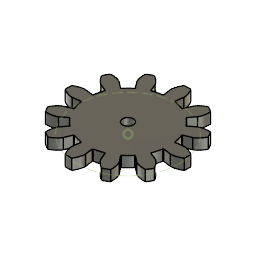
klenn final 1 (Autodesk Fusion 360 archive; units mm, degrees)
design "klenn part_Spur Gear 12 teeth"
description: Spur Gear; Module: 4.0; Num Teeth: 12; Pressure Angle: 14.500000000000002; Backlash: 0.00 mm
part number: 2026-03-30-23-41-15-883
Autodesk Fusion 360 part; units mm, degrees
sketch "Base Circle" plane through (0, 0, 0) normal (0, 0, 1) x (1, 0, 0)
  circle A0 centre (0, 0) radius 19.372
  circle A1 centre (0, 0) radius 2.5
extrude "Extrude1" add sketch "Base Circle" along normal blind 5
sketch "Gear Tooth" plane through (0, 0, 0) normal (0, 0, 1) x (1, 0, 0)
  spline S0 degree 5 poles (23.0196, -3.1605) (23.0336, -3.1625) (23.0617, -3.1659) (23.1038, -3.1698) (23.1603, -3.1727) (23.231, -3.173) (23.302, -3.171) (23.373, -3.1677) (23.4442, -3.1635) (23.5153, -3.1589) (23.5865, -3.1536) (23.6578, -3.1477) (23.7291, -3.1407) (23.8004, -3.1326) (23.8718, -3.1234) (23.9433, -3.1131) (24.0147, -3.102) (24.0862, -3.0901) (24.1576, -3.0775) (24.2291, -3.0643) (24.3005, -3.0505) (24.372, -3.036) (24.4435, -3.0208) (24.5149, -3.0049) (24.5863, -2.9883) (24.6577, -2.9711) (24.7291, -2.9531) (24.8005, -2.9346) (24.8719, -2.9155) (24.9432, -2.8958) (25.0145, -2.8755) (25.0858, -2.8547) (25.157, -2.8332) (25.2282, -2.8112) (25.2993, -2.7887) (25.3705, -2.7656) (25.4415, -2.7419) (25.5126, -2.7177) (25.5835, -2.6929) (25.6545, -2.6677) (25.7254, -2.6419) (25.7962, -2.6156) (25.867, -2.5888) (25.9377, -2.5615) (26.0083, -2.5337) (26.0789, -2.5054) (26.1495, -2.4766) (26.2199, -2.4473) (26.2903, -2.4175) (26.3607, -2.3873) (26.4309, -2.3566) (26.5011, -2.3254) (26.5713, -2.2937) (26.6413, -2.2616) (26.7113, -2.229) (26.7812, -2.196) (26.851, -2.1625) (26.9207, -2.1285) (26.9904, -2.0942) (27.06, -2.0593) (27.1295, -2.024) (27.1989, -1.9883) (27.2682, -1.9522) (27.3374, -1.9156) (27.4065, -1.8786) (27.4756, -1.8411) (27.5445, -1.8033) (27.6134, -1.765) (27.6821, -1.7263) (27.7508, -1.6872) (27.8193, -1.6476) (27.8741, -1.6156) (27.9151, -1.5915) (27.9424, -1.5753) (27.9561, -1.5672) knots 0 0 0 0 0 0 0.01428571 0.02857143 0.04285714 0.05714286 0.07142857 0.08571429 0.1 0.11428571 0.12857143 0.14285714 0.15714286 0.17142857 0.18571429 0.2 0.21428571 0.22857143 0.24285714 0.25714286 0.27142857 0.28571429 0.3 0.31428571 0.32857143 0.34285714 0.35714286 0.37142857 0.38571429 0.4 0.41428571 0.42857143 0.44285714 0.45714286 0.47142857 0.48571429 0.5 0.51428571 0.52857143 0.54285714 0.55714286 0.57142857 0.58571429 0.6 0.61428571 0.62857143 0.64285714 0.65714286 0.67142857 0.68571429 0.7 0.71428571 0.72857143 0.74285714 0.75714286 0.77142857 0.78571429 0.8 0.81428571 0.82857143 0.84285714 0.85714286 0.87142857 0.88571429 0.9 0.91428571 0.92857143 0.94285714 0.95714286 0.97142857 0.98571429 1 1 1 1 1 1
  spline S1 degree 5 poles (23.0196, 3.1605) (23.0336, 3.1625) (23.0617, 3.1659) (23.1038, 3.1698) (23.1603, 3.1727) (23.231, 3.173) (23.302, 3.171) (23.373, 3.1677) (23.4442, 3.1635) (23.5153, 3.1589) (23.5865, 3.1536) (23.6578, 3.1477) (23.7291, 3.1407) (23.8004, 3.1326) (23.8718, 3.1234) (23.9433, 3.1131) (24.0147, 3.102) (24.0862, 3.0901) (24.1576, 3.0775) (24.2291, 3.0643) (24.3005, 3.0505) (24.372, 3.036) (24.4435, 3.0208) (24.5149, 3.0049) (24.5863, 2.9883) (24.6577, 2.9711) (24.7291, 2.9531) (24.8005, 2.9346) (24.8719, 2.9155) (24.9432, 2.8958) (25.0145, 2.8755) (25.0858, 2.8547) (25.157, 2.8332) (25.2282, 2.8112) (25.2993, 2.7887) (25.3705, 2.7656) (25.4415, 2.7419) (25.5126, 2.7177) (25.5835, 2.6929) (25.6545, 2.6677) (25.7254, 2.6419) (25.7962, 2.6156) (25.867, 2.5888) (25.9377, 2.5615) (26.0083, 2.5337) (26.0789, 2.5054) (26.1495, 2.4766) (26.2199, 2.4473) (26.2903, 2.4175) (26.3607, 2.3873) (26.4309, 2.3566) (26.5011, 2.3254) (26.5713, 2.2937) (26.6413, 2.2616) (26.7113, 2.229) (26.7812, 2.196) (26.851, 2.1625) (26.9207, 2.1285) (26.9904, 2.0942) (27.06, 2.0593) (27.1295, 2.024) (27.1989, 1.9883) (27.2682, 1.9522) (27.3374, 1.9156) (27.4065, 1.8786) (27.4756, 1.8411) (27.5445, 1.8033) (27.6134, 1.765) (27.6821, 1.7263) (27.7508, 1.6872) (27.8193, 1.6476) (27.8741, 1.6156) (27.9151, 1.5915) (27.9424, 1.5753) (27.9561, 1.5672) knots 0 0 0 0 0 0 0.01428571 0.02857143 0.04285714 0.05714286 0.07142857 0.08571429 0.1 0.11428571 0.12857143 0.14285714 0.15714286 0.17142857 0.18571429 0.2 0.21428571 0.22857143 0.24285714 0.25714286 0.27142857 0.28571429 0.3 0.31428571 0.32857143 0.34285714 0.35714286 0.37142857 0.38571429 0.4 0.41428571 0.42857143 0.44285714 0.45714286 0.47142857 0.48571429 0.5 0.51428571 0.52857143 0.54285714 0.55714286 0.57142857 0.58571429 0.6 0.61428571 0.62857143 0.64285714 0.65714286 0.67142857 0.68571429 0.7 0.71428571 0.72857143 0.74285714 0.75714286 0.77142857 0.78571429 0.8 0.81428571 0.82857143 0.84285714 0.85714286 0.87142857 0.88571429 0.9 0.91428571 0.92857143 0.94285714 0.95714286 0.97142857 0.98571429 1 1 1 1 1 1
  arc A0 (27.9561, -1.5672) -> (27.9561, 1.5672) centre (0, 0) ccw
  line L0 (19.182, -2.6336) -> (23.0196, -3.1605)
  line L1 (19.182, 2.6336) -> (23.0196, 3.1605)
  line L2 (19.182, -2.6336) -> (19.182, 2.6336)
  point P0 (23.362, -3.168)
  point P1 (23.7088, -3.1425)
  point P2 (24.0583, -3.0946)
  point P3 (24.4097, -3.0279)
  point P4 (24.7627, -2.9443)
  point P5 (25.1168, -2.8453)
  point P6 (25.4717, -2.7315)
  point P7 (25.8272, -2.6038)
  point P8 (26.1829, -2.4626)
  point P9 (26.5385, -2.3084)
  point P10 (26.8939, -2.1415)
  point P11 (27.2488, -1.9622)
  point P12 (27.6029, -1.7707)
  point P13 (23.362, 3.168)
  point P14 (23.7088, 3.1425)
  point P15 (24.0583, 3.0946)
  point P16 (24.4097, 3.0279)
  point P17 (24.7627, 2.9443)
  point P18 (25.1168, 2.8453)
  point P19 (25.4717, 2.7315)
  point P20 (25.8272, 2.6038)
  point P21 (26.1829, 2.4626)
  point P22 (26.5385, 2.3084)
  point P23 (26.8939, 2.1415)
  point P24 (27.2488, 1.9622)
  point P25 (27.6029, 1.7707)
extrude "Extrude2" add sketch "Gear Tooth" along normal blind 5
fillet "Fillet1" radius 0.2 2 edges at (19.192, -2.635, 2.5) (19.192, 2.635, 2.5)
pattern_circular "C-Pattern1" count 12 over 360 about axis through (0, 0, 0) along (0, 0, 1) of "Extrude2", "Fillet1"
sketch "Diametrial Pitch Circle" plane through (0, 0, 0) normal (0, 0, 1) x (1, 0, 0)
  circle A0 centre (0, 0) radius 24 construction

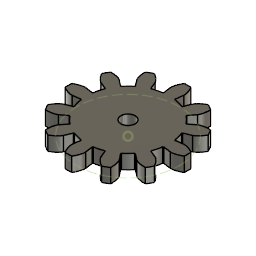
design "klenn part_Spur Gear 12 teeth (1)"
description: Spur Gear; Module: 3.0; Num Teeth: 12; Pressure Angle: 14.500000000000002; Backlash: 0.00 mm
part number: 2026-03-30-23-48-04-964
Autodesk Fusion 360 part; units mm, degrees
sketch "Base Circle" plane through (0, 0, 0) normal (0, 0, 1) x (1, 0, 0)
  circle A0 centre (0, 0) radius 14.529
  circle A1 centre (0, 0) radius 2.5
extrude "Extrude1" add sketch "Base Circle" along normal blind 5
sketch "Gear Tooth" plane through (0, 0, 0) normal (0, 0, 1) x (1, 0, 0)
  spline S0 degree 5 poles (17.2647, -2.3704) (17.2752, -2.3718) (17.2962, -2.3744) (17.3277, -2.3773) (17.3699, -2.3795) (17.4228, -2.3798) (17.4758, -2.3783) (17.529, -2.3758) (17.5822, -2.3727) (17.6355, -2.3692) (17.6887, -2.3653) (17.7421, -2.3609) (17.7954, -2.3557) (17.8488, -2.3497) (17.9023, -2.3428) (17.9557, -2.3351) (18.0092, -2.3268) (18.0627, -2.3179) (18.1162, -2.3085) (18.1697, -2.2986) (18.2232, -2.2883) (18.2768, -2.2775) (18.3303, -2.2661) (18.3838, -2.2542) (18.4373, -2.2418) (18.4908, -2.2289) (18.5443, -2.2155) (18.5978, -2.2016) (18.6513, -2.1873) (18.7048, -2.1726) (18.7582, -2.1574) (18.8116, -2.1418) (18.865, -2.1258) (18.9184, -2.1093) (18.9718, -2.0924) (19.0251, -2.0751) (19.0784, -2.0573) (19.1317, -2.0392) (19.1849, -2.0207) (19.2381, -2.0017) (19.2913, -1.9824) (19.3445, -1.9627) (19.3976, -1.9426) (19.4506, -1.9222) (19.5037, -1.9013) (19.5566, -1.8801) (19.6096, -1.8585) (19.6625, -1.8365) (19.7153, -1.8142) (19.7681, -1.7915) (19.8209, -1.7684) (19.8736, -1.745) (19.9263, -1.7213) (19.9789, -1.6972) (20.0314, -1.6727) (20.084, -1.6479) (20.1364, -1.6228) (20.1888, -1.5973) (20.2411, -1.5714) (20.2934, -1.5453) (20.3456, -1.5188) (20.3978, -1.492) (20.4499, -1.4648) (20.5019, -1.4373) (20.5539, -1.4095) (20.6058, -1.3814) (20.6576, -1.3529) (20.7093, -1.3241) (20.761, -1.295) (20.8127, -1.2656) (20.8642, -1.2359) (20.9054, -1.2118) (20.9362, -1.1937) (20.9568, -1.1815) (20.9671, -1.1754) knots 0 0 0 0 0 0 0.01428571 0.02857143 0.04285714 0.05714286 0.07142857 0.08571429 0.1 0.11428571 0.12857143 0.14285714 0.15714286 0.17142857 0.18571429 0.2 0.21428571 0.22857143 0.24285714 0.25714286 0.27142857 0.28571429 0.3 0.31428571 0.32857143 0.34285714 0.35714286 0.37142857 0.38571429 0.4 0.41428571 0.42857143 0.44285714 0.45714286 0.47142857 0.48571429 0.5 0.51428571 0.52857143 0.54285714 0.55714286 0.57142857 0.58571429 0.6 0.61428571 0.62857143 0.64285714 0.65714286 0.67142857 0.68571429 0.7 0.71428571 0.72857143 0.74285714 0.75714286 0.77142857 0.78571429 0.8 0.81428571 0.82857143 0.84285714 0.85714286 0.87142857 0.88571429 0.9 0.91428571 0.92857143 0.94285714 0.95714286 0.97142857 0.98571429 1 1 1 1 1 1
  spline S1 degree 5 poles (17.2647, 2.3704) (17.2752, 2.3718) (17.2962, 2.3744) (17.3277, 2.3773) (17.3699, 2.3795) (17.4228, 2.3798) (17.4758, 2.3783) (17.529, 2.3758) (17.5822, 2.3727) (17.6355, 2.3692) (17.6887, 2.3653) (17.7421, 2.3609) (17.7954, 2.3557) (17.8488, 2.3497) (17.9023, 2.3428) (17.9557, 2.3351) (18.0092, 2.3268) (18.0627, 2.3179) (18.1162, 2.3085) (18.1697, 2.2986) (18.2232, 2.2883) (18.2768, 2.2775) (18.3303, 2.2661) (18.3838, 2.2542) (18.4373, 2.2418) (18.4908, 2.2289) (18.5443, 2.2155) (18.5978, 2.2016) (18.6513, 2.1873) (18.7048, 2.1726) (18.7582, 2.1574) (18.8116, 2.1418) (18.865, 2.1258) (18.9184, 2.1093) (18.9718, 2.0924) (19.0251, 2.0751) (19.0784, 2.0573) (19.1317, 2.0392) (19.1849, 2.0207) (19.2381, 2.0017) (19.2913, 1.9824) (19.3445, 1.9627) (19.3976, 1.9426) (19.4506, 1.9222) (19.5037, 1.9013) (19.5566, 1.8801) (19.6096, 1.8585) (19.6625, 1.8365) (19.7153, 1.8142) (19.7681, 1.7915) (19.8209, 1.7684) (19.8736, 1.745) (19.9263, 1.7213) (19.9789, 1.6972) (20.0314, 1.6727) (20.084, 1.6479) (20.1364, 1.6228) (20.1888, 1.5973) (20.2411, 1.5714) (20.2934, 1.5453) (20.3456, 1.5188) (20.3978, 1.492) (20.4499, 1.4648) (20.5019, 1.4373) (20.5539, 1.4095) (20.6058, 1.3814) (20.6576, 1.3529) (20.7093, 1.3241) (20.761, 1.295) (20.8127, 1.2656) (20.8642, 1.2359) (20.9054, 1.2118) (20.9362, 1.1937) (20.9568, 1.1815) (20.9671, 1.1754) knots 0 0 0 0 0 0 0.01428571 0.02857143 0.04285714 0.05714286 0.07142857 0.08571429 0.1 0.11428571 0.12857143 0.14285714 0.15714286 0.17142857 0.18571429 0.2 0.21428571 0.22857143 0.24285714 0.25714286 0.27142857 0.28571429 0.3 0.31428571 0.32857143 0.34285714 0.35714286 0.37142857 0.38571429 0.4 0.41428571 0.42857143 0.44285714 0.45714286 0.47142857 0.48571429 0.5 0.51428571 0.52857143 0.54285714 0.55714286 0.57142857 0.58571429 0.6 0.61428571 0.62857143 0.64285714 0.65714286 0.67142857 0.68571429 0.7 0.71428571 0.72857143 0.74285714 0.75714286 0.77142857 0.78571429 0.8 0.81428571 0.82857143 0.84285714 0.85714286 0.87142857 0.88571429 0.9 0.91428571 0.92857143 0.94285714 0.95714286 0.97142857 0.98571429 1 1 1 1 1 1
  arc A0 (20.9671, -1.1754) -> (20.9671, 1.1754) centre (0, 0) ccw
  line L0 (14.3841, -1.9749) -> (17.2647, -2.3704)
  line L1 (14.3841, 1.9749) -> (17.2647, 2.3704)
  line L2 (14.3841, -1.9749) -> (14.3841, 1.9749)
  point P0 (17.5215, -2.376)
  point P1 (17.7816, -2.3569)
  point P2 (18.0437, -2.321)
  point P3 (18.3073, -2.2709)
  point P4 (18.572, -2.2083)
  point P5 (18.8376, -2.1339)
  point P6 (19.1038, -2.0486)
  point P7 (19.3704, -1.9529)
  point P8 (19.6371, -1.847)
  point P9 (19.9039, -1.7313)
  point P10 (20.1704, -1.6062)
  point P11 (20.4366, -1.4717)
  point P12 (20.7022, -1.328)
  point P13 (17.5215, 2.376)
  point P14 (17.7816, 2.3569)
  point P15 (18.0437, 2.321)
  point P16 (18.3073, 2.2709)
  point P17 (18.572, 2.2083)
  point P18 (18.8376, 2.1339)
  point P19 (19.1038, 2.0486)
  point P20 (19.3704, 1.9529)
  point P21 (19.6371, 1.847)
  point P22 (19.9039, 1.7313)
  point P23 (20.1704, 1.6062)
  point P24 (20.4366, 1.4717)
  point P25 (20.7022, 1.328)
extrude "Extrude2" add sketch "Gear Tooth" along normal blind 5
fillet "Fillet1" radius 0.2 2 edges at (14.394, -1.9763, 2.5) (14.394, 1.9763, 2.5)
pattern_circular "C-Pattern1" count 12 over 360 about axis through (0, 0, 0) along (0, 0, 1) of "Extrude2", "Fillet1"
sketch "Diametrial Pitch Circle" plane through (0, 0, 0) normal (0, 0, 1) x (1, 0, 0)
  circle A0 centre (0, 0) radius 18 construction
